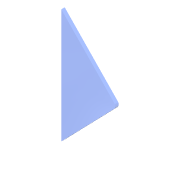
# Autodesk Inventor part: 본체 글라스
Saved by Autodesk Inventor 2020 (Build 240168000, 168)
## iProperties
Created: 2020-06-04
Part Number: 본체 글라스
Material: 일반
Document SubType Name: Modeling
Designer: Miji
Density: 1 g/cm^3
Appearance: 선명 - 파란색
Author: Miji
Autodesk Inventor part; units mm, degrees
ref_plane "YZ Plane" through (0, 0, 0) normal (1, 0, 0) x (0, 1, 0)
ref_plane "XZ Plane" through (0, 0, 0) normal (0, 1, 0) x (-1, 0, 0)
ref_plane "XY Plane" through (0, 0, 0) normal (0, 0, 1) x (1, 0, 0)
sketch "스케치1" plane through (0, 0, 0) normal (0, 0, 1) x (1, 0, 0)
  line L0 (-8.6981, -1.3757) -> (-39.2674, -32.97) projected
  arc A0 (-8.6981, -1.3757) -> (-8.6981, 1.4057) centre (-10.1355, 0.015) ccw projected
  line L1 (-37.7674, -29.2626) -> (-37.7674, 29.2925) projected
  line L2 (-37.7674, 29.2925) -> (-9.7762, 0.3627) projected
  arc A1 (-9.7762, -0.3327) -> (-9.7762, 0.3627) centre (-10.1355, 0.015) ccw projected
  line L3 (-9.7762, -0.3327) -> (-37.7674, -29.2626) projected
  arc A2 (-8.6981, -1.3757) -> (-8.6981, 1.4057) centre (-10.1355, 0.015) ccw projected
  line L4 (-39.2674, 33) -> (-8.6981, 1.4057) projected
  line L5 (-39.2674, -32.97) -> (-39.2674, 33) projected
  line L6 (-8.6981, -1.3757) -> (-39.2674, -32.97) projected
  point P0 (0, 0)
extrude "돌출1" add sketch "스케치1" against normal blind 2 contours L0 L5 L4 A0 | L1 L2 A1 L3
